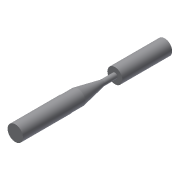
# Autodesk Inventor part: transmission plunger
Saved by Autodesk Inventor 2014 (Build 180170000, 170)
## iProperties
Created: 2014-02-22
Part Number: transmission plunger
Material: Generic
Document SubType Name: Modeling
Designer: Owner
Density: 1 g/cm^3
Appearance: Default
Author: Owner
Autodesk Inventor part; units mm, degrees
sketch "Sketch1" plane through (0, 0, 0) normal (0, 0, 1) x (1, 0, 0)
  circle A0 centre (0, 0) radius 3.937
  dimension "d0" = 7.874
  constraints: 1 centre point
  measures "d0" diameter of A0
extrude "Extrusion1" add sketch "Sketch1" along normal blind 76.2
sketch "Sketch2" plane through (0, 0, 0) normal (0, 0, -1) x (-1, 0, 0)
  circle A0 centre (0, 0) radius 3.937 projected
  circle A1 centre (0, 0) radius 3.81
  dimension "d3" = 7.62
  constraints: 1 centre point, 1 coincident
  measures "d3" diameter of A1
extrude "Extrusion2" cut sketch "Sketch2" against normal blind 50.8
ref_plane "Work Plane1" through (0, 0, 25.4) normal (0, 0, -1) x (-1, 0, 0)
sketch "Sketch3" plane through (0, 0, 25.4) normal (0, 0, -1) x (-1, 0, 0)
  circle A0 centre (0, 0) radius 3.81 projected
  circle A1 centre (0, 0) radius 1.5875
  dimension "d7" = 3.175
  constraints: 1 centre point, 1 coincident
  measures "d7" diameter of A1
ref_plane "Work Plane2" through (0, 0, 31.75) normal (0, 0, -1) x (-1, 0, 0)
ref_plane "Work Plane3" through (0, 0, 44.45) normal (0, 0, -1) x (-1, 0, 0)
sketch "Sketch4" plane through (0, 0, 31.75) normal (0, 0, -1) x (-1, 0, 0)
  circle A0 centre (0, 0) radius 3.81 projected
  circle A1 centre (0, 0) radius 1.5875
  dimension "d10" = 3.175
  constraints: 1 centre point, 1 coincident
  measures "d10" diameter of A1
sketch "Sketch5" plane through (0, 0, 0) normal (0, 1, 0) x (-1, 0, 0)
  line L0 (3.81, 0) -> (3.81, 50.8) projected
  line L1 (-3.81, 0) -> (-3.81, 50.8) projected
  line L2 (5.5118, 31.75) -> (-5.5118, 31.75) projected
  line L3 (5.5118, 25.4) -> (-5.5118, 25.4) projected
  line L4 (3.81, 25.4) -> (1.3426, 25.4)
  line L5 (1.3426, 25.4) -> (1.3426, 31.75)
  line L6 (1.3426, 31.75) -> (3.81, 31.75)
  line L7 (3.81, 31.75) -> (3.81, 25.4)
  line L8 (0, 31.75) -> (0, 25.4) construction
  constraints: 10 end point, 3 midpoint, 2 parallel, 2 perpendicular, 2 point on line, 1 horizontal
revolve "Revolution1" cut sketch "Sketch5" angle 360 about axis through (0, 0, 31.75) along (0, 0, -1) contours L3 L5 L2 L0
sketch "Sketch6" plane through (0, 0, 44.45) normal (0, 0, -1) x (-1, 0, 0)
  circle A0 centre (0, 0) radius 3.81 projected
  circle A1 centre (0, 0) radius 3.937 projected
  line L0 (0, 0) -> (0, 3.81) construction
  constraints: 2 end point, 2 vertical alignment, 2 other
sketch "Sketch8" plane through (0, 0, 0) normal (1, 0, 0) x (0, 1, 0)
  line L0 (5.5118, 31.75) -> (-5.5118, 31.75) projected
  line L1 (5.5118, 44.45) -> (-5.5118, 44.45) projected
  line L2 (1.3249, 31.75) -> (3.8367, 44.45)
  line L3 (0, 31.75) -> (0, 44.45) construction
  line L4 (3.8367, 44.45) -> (3.8367, 31.75)
  constraints: 6 end point, 3 point on line, 2 midpoint, 2 perpendicular
revolve "Revolution2" cut sketch "Sketch8" angle 360 about axis through (0, 0, 31.75) along (0, 0, 1)
body "Solid1"
